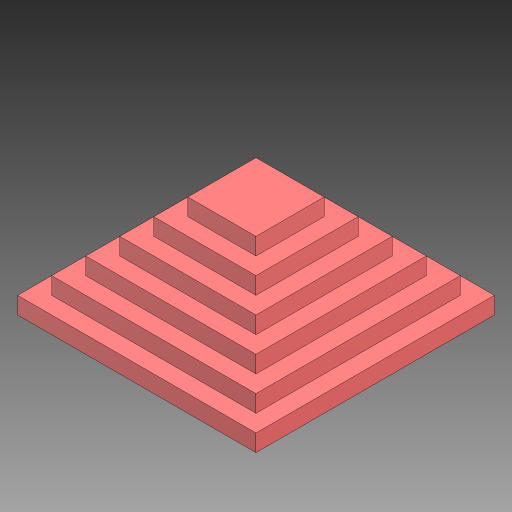
# Autodesk Inventor part: strecha
Saved by Autodesk Inventor 2023 (Build 270158000, 158)
## iProperties
Created: 2022-10-19
Part Number: strecha
Material: Dřevo (dub)
Document SubType Name: Modeling
Designer: zak
Density: 0.76 g/cm^3
Appearance: Hladká – červená
Mass: 1326.59 g
Surface Area: 1438.45 cm^2
Volume: 1745.51 cm^3
Author: zak
Autodesk Inventor part; units mm, degrees
ref_plane "YZ Plane" through (0, 0, 0) normal (1, 0, 0) x (0, 1, 0)
ref_plane "XZ Plane" through (0, 0, 0) normal (0, 1, 0) x (-1, 0, 0)
ref_plane "XY Plane" through (0, 0, 0) normal (0, 0, 1) x (1, 0, 0)
sketch "Náčrt1" plane through (0, 0, 0) normal (0, 1, 0) x (-1, 0, 0)
  line L0 (105, 105) -> (-105, 105)
  line L1 (-105, 105) -> (-105, -105)
  line L2 (-105, -105) -> (105, -105)
  line L3 (105, -105) -> (105, 105)
  line L4 (105, 105) -> (-105, -105) construction
  line L5 (-105, 105) -> (105, -105) construction
  point P0 (0, 0)
  dimension "d0" = 210
  dimension "d1" = 210
  constraints: 12 end point, 2 midpoint, 2 parallel, 1 horizontal, 1 perpendicular
  measures "d0" distance of L2.end L1.end
  measures "d1" distance of L1.end L0.end
extrude "Vysunutí1" add sketch "Náčrt1" along normal blind 15
sketch "Náčrt2" plane through (0, 15, 0) normal (0, 1, 0) x (1, 0, 0)
  line L0 (90, -90) -> (-90, -90)
  line L1 (-90, -90) -> (-90, 90)
  line L2 (-90, 90) -> (90, 90)
  line L3 (90, 90) -> (90, -90)
  line L4 (90, -90) -> (-90, 90) construction
  line L5 (-90, -90) -> (90, 90) construction
  point P0 (0, 0)
  dimension "d4" = 180
  dimension "d5" = 180
  constraints: 12 end point, 2 midpoint, 2 parallel, 1 horizontal, 1 perpendicular
  measures "d4" distance of L1.end L2.end
  measures "d5" distance of L0.end L1.end
extrude "Vysunutí2" add sketch "Náčrt2" along normal blind 15
sketch "Náčrt3" plane through (0, 30, 0) normal (0, 1, 0) x (1, 0, 0)
  line L0 (75, -75) -> (-75, -75)
  line L1 (-75, -75) -> (-75, 75)
  line L2 (-75, 75) -> (75, 75)
  line L3 (75, 75) -> (75, -75)
  line L4 (75, -75) -> (-75, 75) construction
  line L5 (-75, -75) -> (75, 75) construction
  point P0 (0, 0)
  dimension "d8" = 150
  dimension "d9" = 150
  constraints: 12 end point, 2 midpoint, 2 parallel, 1 horizontal, 1 perpendicular
  measures "d8" distance of L1.end L2.end
  measures "d9" distance of L0.end L1.end
extrude "Vysunutí3" add sketch "Náčrt3" along normal blind 15
sketch "Náčrt4" plane through (0, 45, 0) normal (0, 1, 0) x (1, 0, 0)
  line L0 (60, -60) -> (-60, -60)
  line L1 (-60, -60) -> (-60, 60)
  line L2 (-60, 60) -> (60, 60)
  line L3 (60, 60) -> (60, -60)
  line L4 (60, -60) -> (-60, 60) construction
  line L5 (-60, -60) -> (60, 60) construction
  point P0 (0, 0)
  dimension "d12" = 120
  dimension "d13" = 120
  constraints: 12 end point, 2 midpoint, 2 parallel, 1 horizontal, 1 perpendicular
  measures "d12" distance of L1.end L2.end
  measures "d13" distance of L0.end L1.end
extrude "Vysunutí4" add sketch "Náčrt4" along normal blind 15
sketch "Náčrt5" plane through (0, 60, 0) normal (0, 1, 0) x (1, 0, 0)
  line L0 (45, -45) -> (-45, -45)
  line L1 (-45, -45) -> (-45, 45)
  line L2 (-45, 45) -> (45, 45)
  line L3 (45, 45) -> (45, -45)
  line L4 (45, -45) -> (-45, 45) construction
  line L5 (-45, -45) -> (45, 45) construction
  point P0 (0, 0)
  dimension "d16" = 90
  dimension "d17" = 90
  constraints: 12 end point, 2 midpoint, 2 parallel, 1 horizontal, 1 perpendicular
  measures "d16" distance of L1.end L2.end
  measures "d17" distance of L0.end L1.end
extrude "Vysunutí5" add sketch "Náčrt5" along normal blind 15
sketch "Náčrt7" plane through (0, 75, 0) normal (0, 1, 0) x (1, 0, 0)
  line L0 (-30, 30) -> (30, 30)
  line L1 (30, 30) -> (30, -30)
  line L2 (30, -30) -> (-30, -30)
  line L3 (-30, -30) -> (-30, 30)
  line L4 (-30, 30) -> (30, -30) construction
  line L5 (30, 30) -> (-30, -30) construction
  point P0 (0, 0)
  dimension "d20" = 60
  dimension "d21" = 60
  constraints: 12 end point, 2 midpoint, 2 parallel, 1 horizontal, 1 perpendicular
  measures "d20" distance of L1.end L2.end
  measures "d21" distance of L0.end L1.end
extrude "Vysunutí6" add sketch "Náčrt7" along normal blind 15
sketch "Náčrt8" plane through (0, 0, 0) normal (0, -1, 0) x (1, 0, 0)
  line L0 (-55, -55) -> (55, -55)
  line L1 (55, -55) -> (55, 55)
  line L2 (55, 55) -> (-55, 55)
  line L3 (-55, 55) -> (-55, -55)
  line L4 (-55, -55) -> (55, 55) construction
  line L5 (55, -55) -> (-55, 55) construction
  point P0 (0, 0)
  dimension "d24" = 110
  dimension "d25" = 110
  constraints: 12 end point, 2 midpoint, 2 parallel, 1 horizontal, 1 perpendicular
  measures "d24" distance of L2.end L1.end
  measures "d25" distance of L0.end L1.end
extrude "Vysunutí7" cut sketch "Náčrt8" against normal blind 10
sketch "Náčrt9" plane through (0, 0, 0) normal (0, -1, 0) x (1, 0, 0)
  line L0 (55, 55) -> (55, -55) projected
  line L1 (55, -49.75) -> (65, -49.75)
  line L2 (65, -49.75) -> (65, -39.75)
  line L3 (65, -39.75) -> (55, -39.75)
  line L4 (55, -39.75) -> (55, -49.75)
  line L5 (55, -55) -> (-55, -55) projected
  point P0 (0, 0)
  dimension "d28" = 10
  dimension "d29" = 10
  dimension "d30" = 5.25
  constraints: 8 end point, 2 parallel, 1 horizontal, 1 perpendicular, 1 point on line
  measures "d28" distance of L3.end L2.end
  measures "d29" distance of L2.end L1.end
  measures "d30" distance between parallel lines of L5 L1
extrude "Vysunutí8" cut sketch "Náčrt9" against normal blind 20
sketch "Náčrt10" plane through (0, 10, 0) normal (0, -1, 0) x (1, 0, 0)
  line L0 (55, -39.75) -> (55, -49.75) projected
  line L1 (55, -49.75) -> (-2.5, -49.75)
  line L2 (-2.5, -49.75) -> (-2.5, -39.75)
  line L3 (-2.5, -39.75) -> (55, -39.75)
  line L4 (55, -39.75) -> (55, -49.75)
  line L5 (-2.5, -49.75) -> (2.5, -49.75)
  line L6 (2.5, -49.75) -> (2.5, 5)
  line L7 (2.5, 5) -> (-2.5, 5)
  line L8 (-2.5, 5) -> (-2.5, -49.75)
  point P0 (0, 0)
  point P1 (2.5, -39.75)
  dimension "d33" = 57.5
  dimension "d34" = 5
  dimension "d35" = 54.75
  constraints: 16 end point, 4 parallel, 2 horizontal, 2 perpendicular
  measures "d33" distance of L2.end L3.end
  measures "d34" distance of L7.end L6.end
  measures "d35" distance of L6.end L5.end
extrude "Vysunutí9" cut sketch "Náčrt10" against normal blind 10
